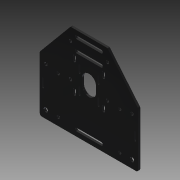
# Autodesk Inventor part: S2_mm
Saved by Autodesk Inventor 2014 (Build 180170000, 170)
## iProperties
Company: www.shapeoko.com
Created: 2011-08-17
Part Number: S2_mm
Material: Steel, Mild
Document SubType Name: Modeling
Designer: ERF
Mass: 471.928 g
Surface Area: 423.918 cm^2
Volume: 60.0418 cm^3
Density: 7.86 g/cm^3
Project: ShapeOko
Checked By: ERF
Catalog Web Link: www.shapeoko.com/
Description: 160mm x 150mm x 10ga, motor mount plate
Vendor: custom
Stock Number: S2_MM
Appearance: Lacquer - Black
Title: Motor Mounting Plate
Subject: Shapeoko v2.0
Author: ERF
Autodesk Inventor part; units mm, degrees
ref_plane "YZ Plane" through (0, 0, 0) normal (1, 0, 0) x (0, 1, 0)
ref_plane "XZ Plane" through (0, 0, 0) normal (0, 1, 0) x (-1, 0, 0)
ref_plane "XY Plane" through (0, 0, 0) normal (0, 0, 1) x (1, 0, 0)
sketch "Sketch1" plane through (0, 0, 0) normal (0, 0, 1) x (1, 0, 0)
  line L0 (10.9384, 8.2044) -> (170.9384, 8.2044)
  line L1 (170.9384, 8.2044) -> (170.9384, 98.2044)
  line L2 (10.9384, 98.2044) -> (10.9384, 8.2044)
  line L3 (10.9384, 98.2044) -> (60.9384, 158.2044)
  line L4 (60.9384, 158.2044) -> (120.9384, 158.2044)
  line L5 (120.9384, 158.2044) -> (170.9384, 98.2044)
  dimension "d0" = 160
  dimension "d4" = 60
  dimension "d5" = 50
  dimension "d6" = 90
  dimension "d7" = 90
  dimension "d8" = 150
  constraints: 12 end point, 2 perpendicular, 1 horizontal, 1 parallel
  measures "d0" distance of L0.start L0.end
  measures "d4" distance of L3.end L4.end
  measures "d5" horizontal distance of L1.end L4.end
  measures "d6" distance of L0.end L1.end
  measures "d7" distance of L0.start L2.start
  measures "d8" distance between parallel lines of L0 L4
extrude "Extrusion1" add sketch "Sketch1" along normal blind 3.4163
sketch "Sketch2" plane through (0, 0, 3.4163) normal (0, 0, 1) x (1, 0, 0)
  line L0 (10.9384, 8.2044) -> (10.9384, 98.2044) projected
  line L1 (170.9384, 8.2044) -> (10.9384, 8.2044) projected
  circle A0 centre (20.9384, 20.9044) radius 3.57
  circle A1 centre (20.9384, 85.5044) radius 2.625
  dimension "d11" = 7.14
  dimension "d12" = 12.7
  dimension "d13" = 10
  dimension "d14" = 10
  dimension "d15" = 64.6
  dimension "d16" = 5.25
  constraints: 2 centre point
  measures "d11" diameter of A0
  measures "d12" distance from line of L1 A0.centre
  measures "d13" distance from line of L0 A0.centre
  measures "d14" distance from line of L0 A1.centre
  measures "d15" distance of A0.centre A1.centre
  measures "d16" diameter of A1
extrude "wheel_holes" cut sketch "Sketch2" against normal through all
pattern_linear "Rectangular Pattern1" count 2 spacing 140 along (1, 0, 0) of "wheel_holes"
sketch "Sketch3" plane through (0, 0, 3.4163) normal (0, 0, 1) x (1, 0, 0)
  line L0 (10.9384, 8.2044) -> (10.9384, 98.2044) projected
  line L1 (170.9384, 8.2044) -> (10.9384, 8.2044) projected
  arc A0 (79.4384, 85.5044) -> (102.4384, 85.5044) centre (90.9384, 85.5044) ccw
  arc A1 (73.8194, 100.9984) -> (77.0694, 100.9984) centre (75.4444, 100.9984) ccw
  line L2 (170.9384, 98.2044) -> (170.9384, 8.2044) projected
  arc A2 (77.0694, 110.9984) -> (73.8194, 110.9984) centre (75.4444, 110.9984) ccw
  line L3 (77.0694, 110.9984) -> (77.0694, 100.9984)
  line L4 (73.8194, 110.9984) -> (73.8194, 100.9984)
  arc A3 (102.4384, 95.5044) -> (79.4384, 95.5044) centre (90.9384, 95.5044) ccw
  line L5 (79.4384, 95.5044) -> (79.4384, 85.5044)
  line L6 (102.4384, 85.5044) -> (102.4384, 95.5044)
  arc A4 (104.8074, 100.9984) -> (108.0574, 100.9984) centre (106.4324, 100.9984) ccw
  arc A5 (108.0574, 110.9984) -> (104.8074, 110.9984) centre (106.4324, 110.9984) ccw
  line L7 (108.0574, 110.9984) -> (108.0574, 100.9984)
  line L8 (104.8074, 110.9984) -> (104.8074, 100.9984)
  arc A6 (73.8194, 70.0104) -> (77.0694, 70.0104) centre (75.4444, 70.0104) ccw
  arc A7 (77.0694, 80.0104) -> (73.8194, 80.0104) centre (75.4444, 80.0104) ccw
  line L9 (77.0694, 80.0104) -> (77.0694, 70.0104)
  line L10 (73.8194, 80.0104) -> (73.8194, 70.0104)
  arc A8 (104.8074, 70.0104) -> (108.0574, 70.0104) centre (106.4324, 70.0104) ccw
  arc A9 (108.0574, 80.0104) -> (104.8074, 80.0104) centre (106.4324, 80.0104) ccw
  line L11 (108.0574, 80.0104) -> (108.0574, 70.0104)
  line L12 (104.8074, 80.0104) -> (104.8074, 70.0104)
  dimension "d22" = 23
  dimension "d23" = 80
  dimension "d24" = 77.3
  dimension "d33" = 3.25
  dimension "d35" = 64.506
  dimension "d36" = 92.794
  dimension "d105" = 10
  dimension "d106" = 64.506
  dimension "d110" = 3.25
  dimension "d112" = 23
  dimension "d113" = 80
  dimension "d114" = 10
  dimension "d126" = 30.988
  dimension "d129" = 30.988
  dimension "d141" = 10
  constraints: 20 end point, 20 point on circle, 10 centre point, 7 tangent, 1 horizontal, 1 vertical, 30 other
  measures "d22" diameter of A0
  measures "d23" distance from line of L0 A0.centre
  measures "d24" distance from line of L1 A0.centre
  measures "d33" diameter of A1
  measures "d35" distance from line of L0 A1.centre
  measures "d36" distance from line of L1 A1.centre
  measures "d105" distance of A1.centre A2.centre
  measures "d106" distance from line of L0 A2.centre
  measures "d110" diameter of A2
  measures "d112" diameter of A3
  measures "d113" distance from line of L0 A3.centre
  measures "d114" distance of A0.centre A3.centre
  measures "d126" distance of L3.end L7.end
  measures "d129" distance of L3.end L9.end
  measures "d141" distance of L6.start L6.end
extrude "Nema_17" cut sketch "Sketch3" against normal through all
sketch "Sketch4" plane through (0, 0, 3.4163) normal (0, 0, 1) x (1, 0, 0)
  circle A0 centre (160.9384, 85.5044) radius 2.625 projected
  circle A1 centre (20.9384, 85.5044) radius 2.625 projected
  line L0 (10.9384, 8.2044) -> (10.9384, 98.2044) projected
  line L1 (170.9384, 98.2044) -> (170.9384, 8.2044) projected
  circle A2 centre (60.9384, 84.0044) radius 2.625
  circle A3 centre (120.9384, 84.0044) radius 2.625
  dimension "d39" = 50
  dimension "d41" = 5.25
  dimension "d42" = 50
  dimension "d43" = 1.5
  dimension "d44" = 5.25
  dimension "d99" = 1.5
  constraints: 2 centre point
  measures "d39" distance from line of L0 A2.centre
  measures "d41" diameter of A2
  measures "d42" distance from line of L1 A3.centre
  measures "d43" vertical distance of A0.centre A3.centre
  measures "d44" diameter of A3
  measures "d99" vertical distance of A1.centre A2.centre
extrude "Idler_Holes" cut sketch "Sketch4" against normal through all contours A2 | A3
sketch "Sketch5" plane through (0, 0, 3.4163) normal (0, 0, 1) x (1, 0, 0)
  line L0 (60.9384, 158.2044) -> (120.9384, 158.2044) projected
  circle A0 centre (110.9384, 148.2044) radius 2.625
  circle A1 centre (110.9384, 128.2044) radius 2.625
  circle A2 centre (70.9384, 148.2044) radius 2.625
  circle A3 centre (70.9384, 128.2044) radius 2.625
  line L1 (70.9384, 150.8294) -> (110.9384, 150.8294)
  line L2 (110.9384, 145.5794) -> (70.9384, 145.5794)
  line L3 (70.9384, 130.8294) -> (110.9384, 130.8294)
  line L4 (110.9384, 125.5794) -> (70.9384, 125.5794)
  dimension "d47" = 10
  dimension "d48" = 10
  dimension "d49" = 20
  dimension "d50" = 10
  dimension "d51" = 5.25
  dimension "d52" = 5.25
  dimension "d87" = 40
  dimension "d145" = 40
  dimension "d146" = 40
  constraints: 8 end point, 8 point on circle, 6 tangent, 4 centre point, 1 horizontal, 4 other
  measures "d47" distance from line of L0 A0.centre
  measures "d48" horizontal distance of L0.end A0.centre
  measures "d49" distance of A0.centre A1.centre
  measures "d50" horizontal distance of L0.end A1.centre
  measures "d51" diameter of A0
  measures "d52" diameter of A1
  measures "d87" distance of A0.centre A2.centre
  measures "d145" distance of L2.end L2.start
  measures "d146" distance of L4.end L4.start
extrude "x-slot" cut sketch "Sketch5" against normal through all
fillet "Fillet2" radius 3.175 6 edges at (120.9384, 158.2044, 1.7082) (60.9384, 158.2044, 1.7082) (170.9384, 98.2044, 1.7082) (170.9384, 8.2044, 1.7082) (10.9384, 98.2044, 1.7082) (10.9384, 8.2044, 1.7082)
sketch "Sketch7" plane through (0, 0, 0) normal (0, 0, -1) x (-1, 0, 0)
  line L0 (-10.9384, 97.0549) -> (-10.9384, 11.3794) projected
  line L1 (-170.9384, 11.3794) -> (-170.9384, 97.0549) projected
  line L2 (-14.1134, 8.2044) -> (-167.7634, 8.2044) projected
  circle A0 centre (-140.9384, 20.9044) radius 2.625
  circle A1 centre (-40.9384, 20.9044) radius 2.625
  dimension "d68" = 5.25
  dimension "d69" = 12.7
  dimension "d70" = 30
  dimension "d71" = 5.25
  dimension "d72" = 30
  dimension "d73" = 12.7
  constraints: 2 centre point
  measures "d68" diameter of A0
  measures "d69" distance from line of L2 A0.centre
  measures "d70" distance from line of L1 A0.centre
  measures "d71" diameter of A1
  measures "d72" distance from line of L0 A1.centre
  measures "d73" distance from line of L2 A1.centre
extrude "two_plater" cut sketch "Sketch7" against normal through all
pattern_linear "Rectangular Pattern3" count 2 spacing 61.5 along (0, 1, 0) of "two_plater"
sketch "Sketch8" plane through (0, 0, 3.4163) normal (0, 0, 1) x (1, 0, 0)
  line L0 (167.7634, 8.2044) -> (14.1134, 8.2044) projected
  line L1 (10.9384, 11.3794) -> (10.9384, 97.0549) projected
  arc A0 (14.3759, 50.7044) -> (17.5009, 50.7044) centre (15.9384, 50.7044) ccw
  arc A1 (17.5009, 62.7044) -> (14.3759, 62.7044) centre (15.9384, 62.7044) ccw
  line L2 (14.3759, 50.7044) -> (14.3759, 62.7044)
  line L3 (17.5009, 62.7044) -> (17.5009, 50.7044)
  arc A2 (164.3759, 50.7044) -> (167.5009, 50.7044) centre (165.9384, 50.7044) ccw
  arc A3 (167.5009, 62.7044) -> (164.3759, 62.7044) centre (165.9384, 62.7044) ccw
  line L4 (164.3759, 50.7044) -> (164.3759, 62.7044)
  line L5 (167.5009, 62.7044) -> (167.5009, 50.7044)
  point P0 (0, 0)
  dimension "d76" = 3.125
  dimension "d77" = 3.125
  dimension "d78" = 12
  dimension "d79" = 5
  dimension "d80" = 42.5
  dimension "d81" = 3.125
  dimension "d82" = 5
  dimension "d94" = 150
  constraints: 8 end point, 8 point on circle, 4 centre point, 3 tangent, 1 horizontal, 10 other
  measures "d76" diameter of A0
  measures "d77" diameter of A1
  measures "d78" distance of A0.centre A1.centre
  measures "d79" distance from line of L1 A0.centre
  measures "d80" distance from line of L0 A0.centre
  measures "d81" distance of L2.start L3.end
  measures "d82" distance from line of L1 A1.centre
  measures "d94" distance of A0.centre A2.centre
extrude "limit_switches" cut sketch "Sketch8" against normal through all
sketch "Sketch10" plane through (0, 0, 3.4163) normal (0, 0, 1) x (1, 0, 0)
  line L0 (167.7634, 8.2044) -> (14.1134, 8.2044) projected
  line L1 (170.9384, 97.0549) -> (170.9384, 11.3794) projected
  arc A0 (70.9384, 20.8294) -> (70.9384, 15.5794) centre (70.9384, 18.2044) ccw
  arc A1 (110.9384, 15.5794) -> (110.9384, 20.8294) centre (110.9384, 18.2044) ccw
  line L2 (70.9384, 20.8294) -> (110.9384, 20.8294)
  line L3 (110.9384, 15.5794) -> (70.9384, 15.5794)
  point P0 (0, 0)
  dimension "d132" = 5.25
  dimension "d133" = 5.25
  dimension "d134" = 10
  dimension "d135" = 10
  dimension "d136" = 40
  dimension "d137" = 40
  dimension "d138" = 60
  constraints: 4 end point, 4 point on circle, 3 tangent, 2 centre point
  measures "d132" diameter of A0
  measures "d133" diameter of A1
  measures "d134" distance from line of L0 A1.centre
  measures "d135" distance from line of L0 A0.centre
  measures "d136" distance of A1.centre A0.centre
  measures "d137" distance of L2.start L2.end
  measures "d138" distance from line of L1 A1.centre
extrude "Extrusion10" cut sketch "Sketch10" against normal through all
sketch "Sketch11" plane through (0, 0, 3.4163) normal (0, 0, 1) x (1, 0, 0)
  line L0 (62.4255, 158.2044) -> (119.4513, 158.2044) projected
  line L1 (10.9384, 11.3794) -> (10.9384, 97.0549) projected
  circle A0 centre (60.9384, 138.2044) radius 2.625
  circle A1 centre (120.9384, 138.2044) radius 2.625
  point P0 (0, 0)
  dimension "d147" = 5.25
  dimension "d148" = 5.25
  dimension "d149" = 60
  dimension "d150" = 20
  dimension "d151" = 20
  dimension "d152" = 50
  constraints: 2 centre point
  measures "d147" diameter of A0
  measures "d148" diameter of A1
  measures "d149" distance of A0.centre A1.centre
  measures "d150" distance from line of L0 A0.centre
  measures "d151" distance from line of L0 A1.centre
  measures "d152" distance from line of L1 A0.centre
extrude "Extrusion11" cut sketch "Sketch11" against normal through all
sketch "Sketch13" plane through (0, 0, 3.4163) normal (0, 0, 1) x (1, 0, 0)
  line L0 (10.9384, 11.3794) -> (10.9384, 97.0549) projected
  arc A0 (102.4384, 95.5044) -> (79.4384, 95.5044) centre (90.9384, 95.5044) ccw projected
  arc A1 (69.9934, 118.603) -> (64.7015, 119.052) centre (67.3684, 119.0744) ccw
  arc A2 (64.7435, 114.0524) -> (69.9934, 114.0744) centre (67.3684, 114.0744) ccw
  line L1 (69.9934, 118.603) -> (69.9934, 114.0744)
  line L2 (64.7435, 114.0524) -> (64.7015, 119.052)
  point P0 (0, 0)
  dimension "d155" = 5.334
  dimension "d156" = 56.43
  dimension "d157" = 23.57
  dimension "d166" = 5.25
  dimension "d167" = 5
  dimension "d168" = 56.43
  constraints: 4 end point, 4 point on circle, 3 tangent, 2 centre point
  measures "d155" diameter of A1
  measures "d156" distance from line of L0 A1.centre
  measures "d157" horizontal distance of A0.centre A1.centre
  measures "d166" diameter of A2
  measures "d167" distance of A1.centre A2.centre
  measures "d168" distance from line of L0 A2.centre
extrude "Extrusion12" cut sketch "Sketch13" against normal through all
pattern_linear "Rectangular Pattern4" count 2 spacing 47.14 along (1, 0, 0) count 2 spacing 47.14 along (0, -1, 0) of "Extrusion12"
equation "\"d7\" = d6"
equation "\"d35\" = d29"
equation "\"d112\" = d22"
equation "\"d113\" = d23"
equation "\"d42\" = d39"
equation "\"d43\" = d99"
equation "\"d44\" = d41"
equation "\"d50\" = d48"
equation "\"d52\" = d51"
equation "\"d76\" = d77"
equation "\"d82\" = d79"
equation "\"d134\" = d135"
equation "\"d29\" = 64.506"
body "Solid1"
